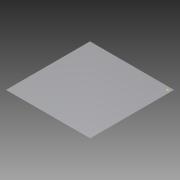
# Autodesk Inventor part: Floor
Saved by Autodesk Inventor 2012 (Build 160160000, 160)
## iProperties
Created: 2009-08-07
Part Number: Floor
Document SubType Name: Modeling
Designer: leefsmp
Density: 1.06 g/cm^3
Mass: 250 g
Surface Area: 5020 cm^2
Volume: 250 cm^3
Material: ABS Plastic
Author: leefsmp
Autodesk Inventor part; units mm, degrees
ref_plane "YZ Plane" through (0, 0, 0) normal (1, 0, 0) x (0, 1, 0)
ref_plane "XZ Plane" through (0, 0, 0) normal (0, 1, 0) x (-1, 0, 0)
ref_plane "XY Plane" through (0, 0, 0) normal (0, 0, 1) x (1, 0, 0)
sketch "Sketch1" plane through (0, 0, 0) normal (0, 0, 1) x (1, 0, 0)
  line L0 (-482.0135, 20.3033) -> (17.9865, 20.3033)
  line L1 (17.9865, 20.3033) -> (17.9865, -479.6967)
  line L2 (17.9865, -479.6967) -> (-482.0135, -479.6967)
  line L3 (-482.0135, -479.6967) -> (-482.0135, 20.3033)
  point P0 (0, 0)
  dimension "x" = 500
  dimension "y" = 500
  constraints: 8 end point, 2 parallel, 1 horizontal, 1 perpendicular
  measures "x" distance of L0.start L0.end
  measures "y" distance of L0.end L1.end
extrude "Extrusion1" add sketch "Sketch1" against normal blind 1
body "Solid1"
